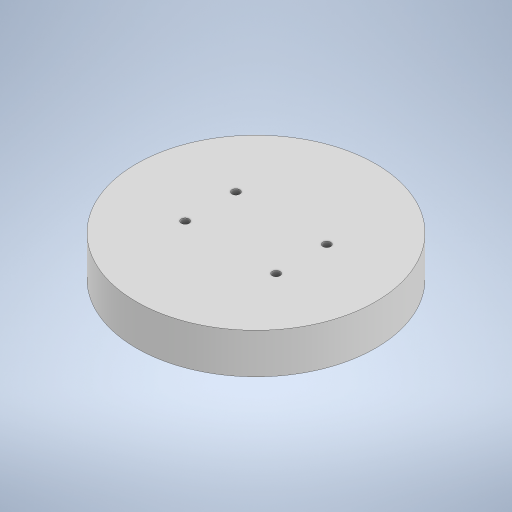
# Autodesk Inventor part: Base_arm_mount
Saved by Autodesk Inventor 2023 (Build 270158000, 158)
## iProperties
Created: 2023-02-09
Part Number: Base_arm_mount
Material: Ogólny
Document SubType Name: Modeling
Designer: kamil
Density: 1 g/cm^3
Appearance: Domyślna
Author: kamil
Autodesk Inventor part; units mm, degrees
ref_plane "YZ Plane" through (0, 0, 0) normal (1, 0, 0) x (0, 1, 0)
ref_plane "XZ Plane" through (0, 0, 0) normal (0, 1, 0) x (-1, 0, 0)
ref_plane "XY Plane" through (0, 0, 0) normal (0, 0, 1) x (1, 0, 0)
sketch "Szkic1" plane through (0, 0, 0) normal (0, 0, 1) x (1, 0, 0)
  line L0 (0, 7.75) -> (46, 7.75)
  line L1 (46, 7.75) -> (46, -7.75)
  line L2 (46, -7.75) -> (42.75, -7.75)
  line L3 (0, -7.75) -> (0, 7.75)
  line L4 (33.25, -7.75) -> (0, -7.75)
  arc A0 (42.75, -7.75) -> (33.25, -7.75) centre (38, -7.75) ccw
  line L5 (0, -10.85) -> (0, 10.85) projected
  line L6 (0, -7.75) -> (33.25, -7.75)
  line L7 (42.75, -7.75) -> (46, -7.75)
  point P0 (0, 0)
  point P1 (0, 0)
  dimension "d0" = 46
  dimension "d1" = 15.5
  dimension "d9" = 38
  dimension "d10" = 4.75
  dimension "d11" = 0
  constraints: 14 end point, 3 parallel, 2 collinear, 2 point on circle, 1 centre point, 1 coincident, 1 horizontal, 1 midpoint, 1 perpendicular
  measures "d0" distance of L1.end L3.start
  measures "d1" distance of L0.end L1.end
  measures "d9" distance of L3.start A0.centre
  measures "d10" radius of A0
  measures "d11" distance from line of L6 A0.centre
revolve "Obrót1" add sketch "Szkic1" angle 360 about axis through (0, -10, 0) along (0, 1, 0)
sketch "Szkic2" plane through (0, -7.75, 0) normal (0, -1, 0) x (1, 0, 0)
  arc A0 (1.3565, -2.1) -> (-1.3565, -2.1) centre (0, 0) ccw
  line L0 (1.3565, -2.1) -> (-1.3565, -2.1)
  point P0 (0, -2.1)
  point P1 (0, 2.5)
  dimension "d5" = 5
  dimension "d15" = 4.6
  constraints: 3 point on circle, 2 end point, 1 centre point, 1 coincident, 1 horizontal, 1 midpoint
  measures "d5" diameter of A0
  measures "d15" distance of point (0, -2.1) point (0, 2.5)
extrude "Wyciągnięcie proste1" cut sketch "Szkic2" against normal blind 13.5
chamfer "Faza1" distance 0.5 angle 45 2 edges at (-42.75, -7.75, 0) (-33.25, -7.75, 0)
sketch "Szkic3" plane through (0, 7.75, 0) normal (0, 1, 0) x (1, 0, 0)
  circle A0 centre (-17.5, -9.75) radius 1.5
  line L0 (64.4, 0) -> (-64.4, 0) projected
  line L1 (0, 64.4) -> (0, -64.4) projected
  circle A1 centre (-17.5, 9.75) radius 1.5
  circle A2 centre (17.5, -9.75) radius 1.5
  circle A3 centre (17.5, 9.75) radius 1.5
  point P0 (0, 0)
  dimension "d16" = 3
  dimension "d17" = 9.75
  dimension "d18" = 17.5
  constraints: 4 centre point, 3 symmetric about line, 3 other
  measures "d16" diameter of A0
  measures "d17" distance from line of L0 A0.centre
  measures "d18" distance from line of L1 A0.centre
extrude "Wyciągnięcie proste2" cut sketch "Szkic3" against normal blind 7
